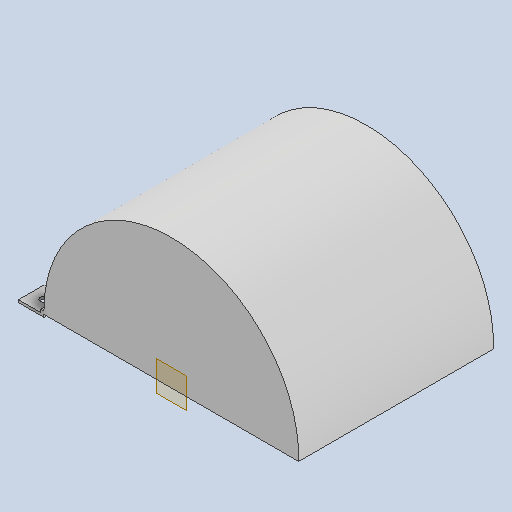
# Autodesk Inventor part: coupol
Saved by Autodesk Inventor 2025 (Build 290162000, 162)
## iProperties
Created: 2025-08-16
Part Number: coupol
Material: Generic
Document SubType Name: Modeling
Designer: Pravoslav
Density: 1 g/cm^3
Appearance: Default
Author: Pravoslav
Autodesk Inventor part; units mm, degrees
ref_plane "YZ Plane" through (0, 0, 0) normal (1, 0, 0) x (0, 1, 0)
ref_plane "XZ Plane" through (0, 0, 0) normal (0, 1, 0) x (-1, 0, 0)
ref_plane "Work Plane1" through (0, 0, 65) normal (0, 0, 1) x (1, 0, 0)
sketch "Sketch1" plane through (0, 0, 65) normal (0, 0, 1) x (1, 0, 0)
  circle A0 centre (0, 0) radius 85
  line L0 (85, 0) -> (-85, 0)
  line L1 (85, 0) -> (-87, 0)
  line L2 (-87, 0) -> (-87, -2)
  line L3 (-87, -2) -> (85, -2)
  line L4 (85, -2) -> (85, 0)
  line L5 (-84.9765, -2) -> (-101.9765, -2)
  line L6 (-101.9765, -2) -> (-101.9765, -3.7)
  line L7 (-101.9765, -3.7) -> (-84.9765, -3.7)
  line L8 (-84.9765, -3.7) -> (-84.9765, -2)
  point P0 (-87, -1)
  point P1 (85, -1)
  point P2 (84.9765, -2)
  dimension "d1" = 170
  dimension "d2" = 2
  dimension "d3" = 0
  dimension "d4" = 172
  dimension "d5" = 17
  dimension "d6" = 1.7
  constraints: 18 end point, 4 parallel, 3 horizontal, 3 point on circle, 2 midpoint, 2 perpendicular, 1 centre point, 1 coincident, 1 point on line
  measures "d1" diameter of A0
  measures "d2" distance between parallel lines of L0 L3
  measures "d3" distance from line of point (0, 0) L0
  measures "d4" distance of point (-87, -1) point (85, -1)
  measures "d5" distance of L7.end L6.end
  measures "d6" distance between parallel lines of L5 L7
extrude "Extrusion1" add sketch "Sketch1" against normal blind 2 contours L0 A0 | A0 L3 L0 | A0 L3 L2 L1 | L8 L7 L6 L5 L3
mirror "Mirror1" about plane through (0, 0, 0) normal (0, 0, 1) of "Extrusion1"
sketch "Sketch2" plane through (0, 0, 63) normal (0, 0, -1) x (-1, 0, 0)
  circle A0 centre (0, 0) radius 83
  arc A1 (85, 0) -> (-84.9765, -2) centre (0, 0) ccw projected
  line L0 (87, 0) -> (87, -2) projected
  line L1 (85, 0) -> (87, 0)
  line L2 (87, 0) -> (87, -2)
  line L3 (87, -2) -> (82.9759, -2)
  line L4 (84.9765, -2) -> (-84.9765, -2) projected
  line L5 (-82.9759, -2) -> (-84.9765, -2)
  circle A2 centre (0, 0) radius 85
  dimension "d9" = 2
  dimension "d10" = 170
  constraints: 8 end point, 2 centre point, 2 coincident, 2 horizontal, 2 point on circle, 1 collinear, 1 perpendicular, 1 point on line
  measures "d9" radial gap between concentric circles of A1 A0
  measures "d10" diameter of A2
extrude "Extrusion2" add sketch "Sketch2" along normal up to surface (126 mm away) contours A0 L4 A1 A2 L3 | A2 L1 L0 L3
sketch "Sketch3" plane through (-101.9765, -3.7, 65) normal (0, -1, 0) x (1, 0, 0)
  line L0 (0, 0) -> (17, 0) projected
  line L1 (0, 0) -> (17, 0)
  line L2 (17, 0) -> (17, -17.5)
  line L3 (17, -17.5) -> (0, -17.5)
  line L4 (0, -17.5) -> (0, 0)
  circle A0 centre (8.25, -8.75) radius 2.5
  point P0 (101.9765, -65)
  dimension "d13" = 17
  dimension "d14" = 17.5
  dimension "d15" = 5
  dimension "d16" = 8.75
  dimension "d17" = 8.75
  constraints: 8 end point, 2 parallel, 1 centre point, 1 horizontal, 1 perpendicular
  measures "d13" distance of L2.end L3.end
  measures "d14" distance of L1.end L2.end
  measures "d15" diameter of A0
  measures "d16" distance from line of L0 A0.centre
  measures "d17" distance from line of A0.centre L2
extrude "Extrusion3" add sketch "Sketch3" against normal up to surface (1.7 mm away)
mirror "Mirror2" about plane through (0, 0, 0) normal (0, 0, 1) of "Extrusion3"
sketch "Sketch4" plane through (-84.9765, -2, 65) normal (0, -1, 0) x (1, 0, 0)
  line L0 (169.9529, 0) -> (169.9529, -130) projected
  line L1 (169.9529, -130) -> (152.4529, -130)
  line L2 (152.4529, -130) -> (152.4529, -112.5)
  line L3 (152.4529, -112.5) -> (169.9529, -112.5)
  line L4 (169.9529, -112.5) -> (169.9529, -130)
  circle A0 centre (161.2029, -121.25) radius 2.5
  point P0 (84.9765, -65)
  dimension "d20" = 17.5
  dimension "d21" = 17.5
  dimension "d22" = 5
  dimension "d23" = 8.75
  dimension "d24" = 8.75
  constraints: 8 end point, 2 parallel, 1 centre point, 1 horizontal, 1 perpendicular
  measures "d20" distance of L2.end L3.end
  measures "d21" distance of L1.end L2.end
  measures "d22" diameter of A0
  measures "d23" distance from line of L0 A0.centre
  measures "d24" distance from line of L1 A0.centre
extrude "Extrusion4" add sketch "Sketch4" against normal blind 2
mirror "Mirror3" about plane through (0, 0, 0) normal (0, 0, 1) of "Extrusion4"
body "Solid1"
